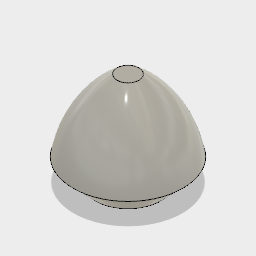
IXS Pod v1 (Autodesk Fusion 360 design; units mm, degrees)
Autodesk Fusion 360 part; units mm, degrees
sketch "Sketch1" plane through (0, 0, 0) normal (1, 0, 0) x (0, 0, -1)
  arc A0 (-9.8991, 64.9629) -> (-50, 0) centre (49.2819, -16.4273) ccw
  line L0 (-9.8991, 64.9629) -> (0, 64.9629)
  line L1 (0, 64.9629) -> (0, -20)
  line L2 (0, -20) -> (-30, -20)
  line L3 (-30, -20) -> (-50, 0)
  constraint horizontal L0
  constraint perpendicular L0 L1
  constraint perpendicular L1 L2
revolve "Revolve1" add sketch "Sketch1" angle 360 about axis through (0, 64.9629, 0) along (0, -1, 0)
